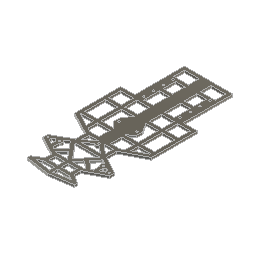
carBodyFrontEnd v1 (Autodesk Fusion 360 design; units mm, degrees)
Autodesk Fusion 360 part; units mm, degrees
(part 1 of 2)
sketch "v0.1" plane through (0, 0, 0) normal (0, 0, 1) x (1, 0, 0)
  line L0 (-45, 50) -> (37, 50)
  line L1 (37, 50) -> (37, 134)
  line L2 (37, 134) -> (-45, 134)
  line L3 (-45, 134) -> (-45, 50)
  line L4 (-69, 50) -> (61, 50)
  line L5 (61, 50) -> (61, -28)
  line L6 (61, -28) -> (-69, -28)
  line L7 (-69, -28) -> (-69, 50)
  line L8 (-30.5, -48) -> (22.5, -48)
  line L9 (22.5, -48) -> (22.5, -65)
  line L10 (22.5, -65) -> (-30.5, -65)
  line L11 (-30.5, -65) -> (-30.5, -48)
  line L12 (-60.5, -82) -> (52.5, -82)
  line L13 (52.5, -82) -> (52.5, -90)
  line L14 (52.5, -90) -> (-60.5, -90)
  line L15 (-60.5, -90) -> (-60.5, -82)
  line L16 (-30.5002, -118) -> (22.4998, -118)
  line L17 (22.4998, -118) -> (22.4998, -107)
  line L18 (22.4998, -107) -> (-30.5002, -107)
  line L19 (-30.5002, -107) -> (-30.5002, -118)
  line L20 (-44.0003, -127.9997) -> (35.9997, -127.9997)
  line L21 (35.9997, -127.9997) -> (35.9997, -132.9997)
  line L22 (35.9997, -132.9997) -> (-44.0003, -132.9997)
  line L23 (-44.0003, -132.9997) -> (-44.0003, -127.9997)
  circle A0 centre (-4.0003, -130.4997) radius 1.6
  circle A1 centre (1.9997, -130.4997) radius 1.6
  circle A2 centre (-10.0003, -130.4997) radius 1.6
  circle A3 centre (-18.0003, -130.4997) radius 1.6
  circle A4 centre (9.9997, -130.4997) radius 1.6
  line L24 (-10.0003, -128.8997) -> (-18.0003, -128.8997)
  line L25 (-10.0003, -132.0997) -> (-18.0003, -132.0997)
  line L26 (1.9997, -128.8997) -> (9.9997, -128.8997)
  line L27 (9.9997, -132.0997) -> (1.9997, -132.0997)
  line L28 (-45, 128.75) -> (-45, 134)
  line L29 (-45, 134) -> (-39.1, 134)
  line L30 (37, 134) -> (31, 134)
  line L31 (31, 134) -> (31, 130)
  line L32 (31, 130) -> (37, 130)
  line L33 (37, 130) -> (37, 134)
  line L34 (-45, 134) -> (-39, 134)
  line L35 (-39, 134) -> (-39, 130)
  line L36 (-39, 130) -> (-45, 130)
  line L37 (-45, 130) -> (-45, 134)
  circle A5 centre (-39, 130) radius 1.6
  circle A6 centre (31, 130) radius 1.6
  circle A7 centre (4.25, 87.9939) radius 1.6
  circle A8 centre (-11.75, 88.0061) radius 1.6
  line L38 (-11.75, 88.0061) -> (-17.75, 88.0107)
  circle A9 centre (-17.75, 88.0107) radius 1.6
  line L39 (4.25, 87.9939) -> (10.25, 87.9939)
  circle A10 centre (10.25, 87.9939) radius 1.6
  line L40 (10.25, 87.9939) -> (20.25, 87.9939)
  circle A11 centre (20.25, 87.9939) radius 1.6
  line L41 (-17.75, 88.0107) -> (-27.75, 88.0184)
  circle A12 centre (-27.75, 88.0184) radius 1.6
  line L42 (-27.7488, 89.6184) -> (-17.7488, 89.6107)
  line L43 (-27.7512, 86.4184) -> (-17.7512, 86.4107)
  line L44 (10.25, 89.5939) -> (20.25, 89.5939)
  line L45 (20.25, 86.3939) -> (10.25, 86.3939)
  line L46 (-69, 50) -> (-57.5, 50)
  line L47 (-57.5, 50) -> (-57.5, 45)
  line L48 (-57.5, 45) -> (-69, 45)
  line L49 (-69, 45) -> (-69, 50)
  circle A13 centre (-57.5, 45) radius 1.6
  line L50 (-57.5, 45) -> (-57.5, 32)
  circle A14 centre (-57.5, 32) radius 1.6
  line L51 (-55.9, 45.0023) -> (-55.9, 32)
  line L52 (-59.1, 45) -> (-59.1, 32)
  line L53 (61, 50) -> (49.5, 50)
  line L54 (49.5, 50) -> (49.5, 45)
  line L55 (49.5, 45) -> (61, 45)
  line L56 (61, 45) -> (61, 50)
  circle A15 centre (49.5, 45) radius 1.6
  line L57 (49.5, 45) -> (49.5, 32)
  circle A16 centre (49.5, 32) radius 1.6
  line L58 (51.1, 45) -> (51.1, 32)
  line L59 (47.9, 32) -> (47.9, 45)
  line L60 (-57.5, 45) -> (-57.5, -26)
  circle A17 centre (-57.5, -26) radius 1.6
  line L61 (49.5, 45) -> (49.5, -26)
  circle A18 centre (49.5, -26) radius 1.6
  circle A19 centre (-4, -51.9) radius 1.6
  circle A20 centre (33.037, -81.135) radius 1.6
  circle A21 centre (-41.033, -81.1414) radius 1.6
  line L62 (22.5, -48) -> (61, -28)
  line L63 (-30.5, -48) -> (-69, -28)
  line L64 (-60.5, -82) -> (-30.5, -65)
  line L65 (22.5, -65) -> (52.5, -82)
  line L66 (22.4998, -107) -> (52.5, -90)
  line L67 (-30.5002, -107) -> (-60.5, -90)
  line L68 (4.25, 87.9939) -> (-11.75, 88.0061)
  line L69 (-4, 134) -> (-3.75, 88)
  line L70 (-44.0003, -127.9997) -> (-30.5002, -118)
  line L71 (35.9997, -127.9997) -> (22.4998, -118)
  line L72 (-4.0003, -132.9997) -> (-4.0003, -138.9997)
  line L73 (-44.0003, -132.9997) -> (-4.0003, -138.9997)
  line L74 (-4.0003, -138.9997) -> (35.9997, -132.9997)
  line L75 (-4.0003, -130.4997) -> (1.9997, -130.4997)
  line L76 (-4.0003, -130.4997) -> (-10.0003, -130.4997)
  line L77 (-4, -65) -> (-4, -83)
  line L78 (-4, -83) -> (-4, -86)
  line L79 (-4, -86) -> (-56, -86)
  line L80 (-4, -86) -> (48, -86)
  circle A22 centre (48, -86) radius 1.1
  circle A23 centre (-56, -86) radius 1.1
  line L81 (20.25, 87.9939) -> (37, 87.9939)
  line L82 (-27.75, 88.0184) -> (-45, 88.0184)
  line L83 (37, 50) -> (24, 50)
  line L84 (24, 50) -> (24, 110)
  line L85 (24, 110) -> (37, 110)
  line L86 (37, 110) -> (37, 50)
  line L87 (-45, 50) -> (-32, 50)
  line L88 (-32, 50) -> (-32, 110)
  line L89 (-32, 110) -> (-45, 110)
  line L90 (-45, 110) -> (-45, 50)
  line L91 (37, 110) -> (31, 110)
  line L92 (31, 110) -> (31, 50)
  line L93 (31, 50) -> (37, 50)
  line L94 (37, 50) -> (37, 110)
  line L95 (-45, 110) -> (-39, 110)
  line L96 (-39, 110) -> (-39, 50)
  line L97 (-39, 50) -> (-45, 50)
  line L98 (-45, 50) -> (-45, 110)
  line L99 (24, 110) -> (27, 110)
  line L100 (27, 110) -> (27, 105)
  line L101 (27, 105) -> (24, 105)
  line L102 (24, 105) -> (24, 110)
  circle A24 centre (27, 105) radius 1.6
  circle A25 centre (27, 88.3333) radius 1.6
  circle A26 centre (27, 71.6667) radius 1.6
  circle A27 centre (27, 55) radius 1.6
  line L103 (-32, 110) -> (-35, 110)
  line L104 (-35, 110) -> (-35, 105)
  line L105 (-35, 105) -> (-32, 105)
  line L106 (-32, 105) -> (-32, 110)
  circle A28 centre (-35, 105) radius 1.6
  circle A29 centre (-35, 88.3333) radius 1.6
  circle A30 centre (-35, 71.6667) radius 1.6
  circle A31 centre (-35, 55) radius 1.6
  line L107 (-69, -28) -> (-49.75, -28)
  line L108 (-49.75, -28) -> (-49.75, -18)
  line L109 (-49.75, -18) -> (-69, -18)
  line L110 (-69, -18) -> (-69, -28)
  line L111 (-69, -18) -> (61, -18)
  line L112 (61, -18) -> (61, 17)
  line L113 (61, 17) -> (-69, 17)
  line L114 (-69, 17) -> (-69, -18)
  line L115 (-69, 17) -> (-55, 17)
  line L116 (-55, 17) -> (-55, 10)
  line L117 (-55, 10) -> (-69, 10)
  line L118 (-69, 10) -> (-69, 17)
  line L119 (61, 17) -> (47, 17)
  line L120 (47, 17) -> (47, 10)
  line L121 (47, 10) -> (61, 10)
  line L122 (61, 10) -> (61, 17)
  circle A32 centre (-55, 10) radius 1.6
  circle A33 centre (-21, 10) radius 1.6
  circle A34 centre (13, 10) radius 1.6
  circle A35 centre (47, 10) radius 1.6
  circle A36 centre (-55, -11) radius 1.6
  circle A37 centre (-21, -11) radius 1.6
  circle A38 centre (13, -11) radius 1.6
  circle A39 centre (47, -11) radius 1.6
  line L123 (-69, 17) -> (61, 17)
  line L124 (61, 17) -> (61, 18)
  line L125 (61, 18) -> (-69, 18)
  line L126 (-69, 18) -> (-69, 17)
  line L127 (61, 18) -> (-69, 18)
  line L128 (-69, 18) -> (-69, 23)
  line L129 (-69, 23) -> (61, 23)
  line L130 (61, 23) -> (61, 18)
  circle A40 centre (18.0038, -78.6409) radius 1.6
  circle A41 centre (18.0038, -78.6409) radius 5
  circle A42 centre (-25.9962, -78.6409) radius 5
  circle A43 centre (-25.9962, -78.6409) radius 1.6
  dimension "d1" = 82
  dimension "d2" = 84
  dimension "d3" = 78
  dimension "d4" = 130
  dimension "d6" = 17
  dimension "d11" = 113
  dimension "d12" = 8
  dimension "d15" = 11
  dimension "d16" = 53
  dimension "d20" = 80
  dimension "d21" = 5
  dimension "d25" = 3.2
  dimension "d29" = 3.2
  dimension "d31" = 3.2
  dimension "d32" = 3.2
  dimension "d35" = 3.2
  dimension "d38" = 6
  dimension "d39" = 4
  dimension "d42" = 6
  dimension "d43" = 4
  dimension "d44" = 3.2
  dimension "d45" = 3.2
  dimension "d53" = 3.2
  dimension "d54" = 3.2
  dimension "d55" = 6
  dimension "d56" = 3.2
  dimension "d58" = 6
  dimension "d59" = 3.2
  dimension "d60" = 10
  dimension "d61" = 3.2
  dimension "d62" = 10
  dimension "d63" = 3.2
  dimension "d64" = 11.5
  dimension "d65" = 3.2
  dimension "d66" = 13
  dimension "d67" = 3.2
  dimension "d68" = 11.5
  dimension "d69" = 5
  dimension "d70" = 5
  dimension "d71" = 3.2
  dimension "d72" = 13
  dimension "d73" = 3.2
  dimension "d74" = 71
  dimension "d75" = 3.2
  dimension "d77" = 71
  dimension "d78" = 3.2
  dimension "d80" = 3.2
  dimension "d83" = 3.2
  dimension "d84" = 3.2
  dimension "d90" = 53
  dimension "d92" = 46
  dimension "d93" = 16
  dimension "d95" = 6
  dimension "d99" = 6
  dimension "d100" = 6
  dimension "d101" = 8
  dimension "d102" = 8
  dimension "d108" = 52
  dimension "d109" = 52
  dimension "d110" = 2.2
  dimension "d111" = 2.2
  dimension "d112" = 13
  dimension "d113" = 60
  dimension "d114" = 13
  dimension "d115" = 60
  dimension "d116" = 60
  dimension "d117" = 6
  dimension "d118" = 60
  dimension "d119" = 3
  dimension "d120" = 5
  dimension "d121" = 3.2
  dimension "d124" = 0
  dimension "d125" = -50
  dimension "d126" = 3
  dimension "d127" = 5
  dimension "d128" = 3.2
  dimension "d131" = 0
  dimension "d132" = -50
  dimension "d133" = 10
  dimension "d134" = 35
  dimension "d135" = 14
  dimension "d136" = 7
  dimension "d137" = 14
  dimension "d138" = 7
  dimension "d139" = 3.2
  dimension "d142" = 102
  dimension "d143" = -21
  dimension "d144" = 1
  dimension "d145" = 130
  dimension "d146" = 5
  dimension "d154" = 3.2
  dimension "d155" = 10
  dimension "d156" = 3.2
  dimension "d157" = 10
  constraint horizontal L0
  constraint vertical L1
  constraint horizontal L2
  constraint vertical L3
  constraint horizontal L4
  constraint vertical L5
  constraint horizontal L6
  constraint vertical L7
  constraint horizontal L8
  constraint vertical L9
  constraint horizontal L10
  constraint vertical L11
  constraint horizontal L12
  constraint vertical L13
  constraint horizontal L14
  constraint vertical L15
  constraint horizontal L16
  constraint vertical L17
  constraint horizontal L18
  constraint vertical L19
  constraint vertical L21
  constraint horizontal L22
  constraint vertical L23
  constraint coincident A2 L24.start
  constraint coincident A3 L24.end
  constraint tangent A3 L24
  constraint coincident A2 L25.start
  constraint coincident A3 L25.end
  constraint tangent A3 L25
  constraint coincident A1 L26.start
  constraint coincident A4 L26.end
  constraint tangent A4 L26
  constraint coincident A4 L27.start
  constraint coincident A1 L27.end
  constraint tangent A1 L27
  constraint vertical L28
  constraint horizontal L29
  constraint horizontal L30
  constraint vertical L31
  constraint horizontal L32
  constraint vertical L33
  constraint horizontal L34
  constraint vertical L35
  constraint horizontal L36
  constraint vertical L37
  constraint coincident L35.end L36.start
  constraint coincident L31.end L32.start
  constraint coincident A8.centre L38.start
  constraint coincident L38.end A9.centre
  constraint coincident A7.centre L39.start
  constraint coincident L39.end A10.centre
  constraint coincident L40.end A11.centre
  constraint coincident L41.end A12.centre
  constraint coincident A12 L42.start
  constraint coincident A9 L42.end
  constraint tangent A9 L42
  constraint coincident A12 L43.start
  constraint coincident A9 L43.end
  constraint tangent A9 L43
  constraint coincident A10 L44.start
  constraint coincident A11 L44.end
  constraint tangent A11 L44
  constraint coincident A11 L45.start
  constraint coincident A10 L45.end
  constraint tangent A10 L45
  constraint horizontal L46
  constraint vertical L47
  constraint horizontal L48
  constraint vertical L49
  constraint coincident L47.end L48.start
  constraint perpendicular L48 L50
  constraint coincident L50.end A14.centre
  constraint coincident A13 L51.start
  constraint coincident A14 L51.end
  constraint tangent A14 L51
  constraint parallel L47 L51
  constraint coincident A13 L52.start
  constraint coincident L48 L52.start
  constraint coincident A14 L52.end
  constraint tangent A14 L52
  constraint horizontal L53
  constraint vertical L54
  constraint horizontal L55
  constraint vertical L56
  constraint coincident L54.end L55.start
  constraint perpendicular L55 L57
  constraint coincident L57.end A16.centre
  constraint coincident A15 L58.start
  constraint coincident L55 L58.start
  constraint coincident A16 L58.end
  constraint tangent A16 L58
  constraint coincident A16 L59.start
  constraint coincident A15 L59.end
  constraint tangent A15 L59
  constraint parallel L50 L60
  constraint coincident L60.end A17.centre
  constraint perpendicular L55 L61
  constraint coincident L61.end A18.centre
  constraint midpoint L2 L69.start
  constraint midpoint L68 L69.end
  constraint tangent A10 L44
  constraint tangent A11 L45
  constraint tangent A12 L42
  constraint tangent A12 L43
  constraint midpoint L22 L72.start
  constraint perpendicular L22 L72
  constraint coincident A0.centre L75.start
  constraint coincident A1.centre L75.end
  constraint coincident A2.centre L76.end
  constraint tangent A2 L24
  constraint tangent A2 L25
  constraint tangent A1 L26
  constraint tangent A4 L27
  constraint midpoint L10 L77.start
  constraint perpendicular L78 L79
  constraint perpendicular L78 L80
  constraint coincident L80.end A22.centre
  constraint coincident L79.end A23.centre
  constraint coincident L1 L81.end
  constraint perpendicular L1 L81
  constraint coincident L3 L82.end
  constraint perpendicular L3 L82
  constraint horizontal L83
  constraint vertical L84
  constraint horizontal L85
  constraint vertical L86
  constraint horizontal L87
  constraint vertical L88
  constraint horizontal L89
  constraint vertical L90
  constraint horizontal L91
  constraint vertical L92
  constraint horizontal L93
  constraint vertical L94
  constraint horizontal L95
  constraint vertical L96
  constraint horizontal L97
  constraint vertical L98
  constraint horizontal L99
  constraint vertical L100
  constraint horizontal L101
  constraint vertical L102
  constraint coincident L100.end L101.start
  constraint horizontal L103
  constraint vertical L104
  constraint horizontal L105
  constraint vertical L106
  constraint coincident L104.end L105.start
  constraint horizontal L107
  constraint vertical L108
  constraint horizontal L109
  constraint vertical L110
  constraint horizontal L111
  constraint vertical L112
  constraint horizontal L113
  constraint vertical L114
  constraint horizontal L115
  constraint vertical L116
  constraint horizontal L117
  constraint vertical L118
  constraint horizontal L119
  constraint vertical L120
  constraint horizontal L121
  constraint vertical L122
  constraint coincident L116.end L117.start
  constraint horizontal L123
  constraint vertical L124
  constraint horizontal L125
  constraint vertical L126
  constraint coincident L5 L124.end
  constraint horizontal L127
  constraint vertical L128
  constraint horizontal L129
  constraint vertical L130
  constraint concentric A40 A41
  constraint concentric A42 A43
  measures "d1" distance of L1.end L2.end
  measures "d2" distance of L0.start L2.end
  measures "d3" distance of L4.end L5.end
  measures "d4" distance of L5.end L6.end
  measures "d6" distance of L8.start L10.end
  measures "d11" distance of L12.start L12.end
  measures "d12" distance of L12.start L14.end
  measures "d15" distance of L16.start L18.end
  measures "d16" distance of L17.end L18.end
  measures "d20" distance of L20.start L20.end
  measures "d21" distance of L20.start L22.end
  measures "d25" diameter of A0
  measures "d29" diameter of A1
  measures "d31" diameter of A2
  measures "d32" diameter of A3
  measures "d35" diameter of A4
  measures "d38" distance of L1.end L30.end
  measures "d39" distance of L1.end L32.end
  measures "d42" distance of L2.end L34.end
  measures "d43" distance of L2.end L36.end
  measures "d44" diameter of A5
  measures "d45" diameter of A6
  measures "d53" diameter of A7
  measures "d54" diameter of A8
  measures "d55" distance of A8.centre L38.end
  measures "d56" diameter of A9
  measures "d58" distance of A7.centre L39.end
  measures "d59" diameter of A10
  measures "d60" distance of L39.end L40.end
  measures "d61" diameter of A11
  measures "d62" distance of L38.end L41.end
  measures "d63" diameter of A12
  measures "d64" distance of L4.start L46.end
  measures "d65" diameter of A13
  measures "d66" distance of L47.end L50.end
  measures "d67" diameter of A14
  measures "d68" distance of L4.end L53.end
  measures "d69" distance of L4.end L55.end
  measures "d70" distance of L4.start L48.end
  measures "d71" diameter of A15
  measures "d72" distance of L54.end L57.end
  measures "d73" diameter of A16
  measures "d74" distance of L47.end L60.end
  measures "d75" diameter of A17
  measures "d77" distance of L54.end L61.end
  measures "d78" diameter of A18
  measures "d80" diameter of A19
  measures "d83" diameter of A20
  measures "d84" diameter of A21
  measures "d90" distance of L8.start L8.end
  measures "d92" vertical distance of L69.start L69.end
  measures "d93" horizontal distance of A7.centre A8.centre
  measures "d95" distance of L72.start L72.end
  measures "d99" distance of A0.centre A1.centre
  measures "d100" distance of A0.centre A2.centre
  measures "d101" distance of L24.start L24.end
  measures "d102" distance of L26.start L26.end
  measures "d108" distance of L78.end L79.end
  measures "d109" distance of L78.end L80.end
  measures "d110" diameter of A22
  measures "d111" diameter of A23
  measures "d112" distance of L0.end L83.end
  measures "d113" distance of L0.end L85.end
  measures "d114" distance of L0.start L87.end
  measures "d115" distance of L0.start L89.end
  measures "d116" distance of L85.end L0.end
  measures "d117" distance of L89.end L95.end
  measures "d118" distance of L89.end L0.start
  measures "d119" distance of L84.end L99.end
  measures "d120" distance of L84.end L101.end
  measures "d121" diameter of A24
  measures "d126" distance of L88.end L103.end
  measures "d127" distance of L88.end L105.end
  measures "d128" diameter of A28
  measures "d133" distance of L6.end L109.end
  measures "d134" distance of L109.end L113.end
  measures "d135" distance of L113.end L115.end
  measures "d136" distance of L113.end L117.end
  measures "d137" distance of L112.end L119.end
  measures "d138" distance of L112.end L121.end
  measures "d139" diameter of A32
  measures "d144" distance of L113.end L125.end
  measures "d145" distance of L124.end L125.end
  measures "d146" distance of L124.end L129.end
  measures "d154" diameter of A40
  measures "d155" diameter of A41
  measures "d156" diameter of A43
  measures "d157" diameter of A42
sketch "v0.2" plane through (0, 0, 0) normal (0, 0, 1) x (1, 0, 0)
  circle A0 centre (-4, -51.9) radius 1.65
  line L0 (-30.5, -48) -> (22.5, -48)
  circle A1 centre (-56, -86) radius 1.1
  line L1 (-69, -28) -> (-69, 50)
  line L2 (61, 50) -> (61, -28)
  line L3 (22.5, -48) -> (61, -28)
  line L4 (-30.5, -65) -> (-30.5, -48)
  line L5 (22.5, -65) -> (-30.5, -65)
  line L6 (22.5, -48) -> (22.5, -65)
  line L7 (-30.5, -48) -> (-69, -28)
  line L8 (35.9997, -127.9997) -> (35.9997, -132.9997)
  circle A2 centre (33.037, -81.135) radius 1.65
  line L9 (-45, 50) -> (37, 50)
  line L10 (-4, -86) -> (48, -86)
  line L11 (-45, 110) -> (-45, 50)
  line L12 (-4.0003, -138.9997) -> (35.9997, -132.9997)
  line L13 (-45, 134) -> (-45, 50)
  line L14 (-69, 50) -> (61, 50)
  line L15 (-4, -86) -> (-56, -86)
  line L16 (-4, -65) -> (-4, -83)
  line L17 (37, 110) -> (37, 50)
  line L18 (24, 50) -> (24, 110)
  line L19 (-39, 50) -> (-45, 50)
  line L20 (31, 110) -> (31, 50)
  line L21 (22.5, -65) -> (52.5, -82)
  line L22 (52.5, -90) -> (-60.5, -90)
  line L23 (-60.5, -82) -> (52.5, -82)
  line L24 (-32, 50) -> (-32, 110)
  line L25 (52.5, -82) -> (52.5, -90)
  line L26 (37, 134) -> (-45, 134)
  line L27 (37, 50) -> (37, 110)
  line L28 (-39, 110) -> (-39, 50)
  line L29 (37, 50) -> (37, 134)
  line L30 (-4, -83) -> (-4, -86)
  line L31 (-60.5, -82) -> (-30.5, -65)
  circle A3 centre (48, -86) radius 1.1
  line L32 (-45, 50) -> (-45, 110)
  line L33 (-32, 110) -> (-45, 110)
  line L34 (-45, 128.75) -> (-45, 134)
  line L35 (-35, 110) -> (-35, 105)
  line L36 (24, 110) -> (37, 110)
  line L37 (31, 50) -> (37, 50)
  line L38 (27, 110) -> (27, 105)
  line L39 (-35, 105) -> (-32, 105)
  line L40 (4.25, 87.9939) -> (10.25, 87.9939)
  circle A4 centre (-35, 55) radius 1.6
  line L41 (-45, 134) -> (-39.1, 134)
  line L42 (-32, 105) -> (-32, 110)
  line L43 (27, 105) -> (24, 105)
  circle A5 centre (27, 88.3333) radius 1.6
  circle A6 centre (27, 105) radius 1.6
  line L44 (-45, 50) -> (-32, 50)
  line L45 (24, 110) -> (27, 110)
  line L46 (-45, 110) -> (-39, 110)
  circle A7 centre (27, 71.6667) radius 1.6
  line L47 (37, 50) -> (24, 50)
  circle A8 centre (27, 55) radius 1.6
  circle A9 centre (-35, 88.3333) radius 1.6
  circle A10 centre (-35, 71.6667) radius 1.6
  line L48 (-32, 110) -> (-35, 110)
  line L49 (37, 110) -> (31, 110)
  circle A11 centre (-35, 105) radius 1.6
  line L50 (24, 105) -> (24, 110)
  line L51 (-60.5, -90) -> (-60.5, -82)
  circle A12 centre (-41.033, -81.1414) radius 1.65
  line L52 (-4.0003, -132.9997) -> (-4.0003, -138.9997)
  line L53 (-44.0003, -132.9997) -> (-4.0003, -138.9997)
  line L54 (-44.0003, -132.9997) -> (-44.0003, -127.9997)
  line L55 (20.4998, -118) -> (-28.5002, -118)
  line L56 (-28.5002, -118) -> (-28.5002, -107)
  line L57 (-28.5002, -107) -> (20.4998, -107)
  line L58 (20.4998, -107) -> (20.4998, -118)
  line L59 (35.9997, -127.9997) -> (20.4998, -118)
  line L60 (-44.0003, -127.9997) -> (-28.5002, -118)
  line L61 (20.4998, -107) -> (52.5, -90)
  line L62 (-28.5002, -107) -> (-60.5, -90)
  line L63 (52.5, -90) -> (44.5, -90)
  line L64 (44.5, -90) -> (44.5, -82)
  line L65 (44.5, -82) -> (52.5, -82)
  line L66 (52.5, -82) -> (52.5, -90)
  line L67 (-60.5, -82) -> (-52.5, -82)
  line L68 (-52.5, -82) -> (-52.5, -90)
  line L69 (-52.5, -90) -> (-60.5, -90)
  line L70 (-60.5, -90) -> (-60.5, -82)
  line L71 (-34.4973, -103.814) -> (-31.6823, -98.5153)
  line L72 (-44.5001, -98.5) -> (-41.6852, -93.2013)
  line L73 (-28.5002, -118) -> (-22.5002, -118)
  line L74 (-22.5002, -118) -> (-22.5002, -107)
  line L75 (-22.5002, -107) -> (-28.5002, -107)
  line L76 (-28.5002, -107) -> (-28.5002, -118)
  line L77 (20.4998, -118) -> (14.4998, -118)
  line L78 (14.4998, -118) -> (14.4998, -107)
  line L79 (14.4998, -107) -> (20.4998, -107)
  line L80 (20.4998, -107) -> (20.4998, -118)
  line L81 (-41.6852, -93.2013) -> (-52.5, -87.4559)
  line L82 (20.4998, -107) -> (-28.5002, -107)
  line L83 (-28.5002, -107) -> (-28.5002, -101)
  line L84 (-28.5002, -101) -> (20.4998, -101)
  line L85 (20.4998, -101) -> (20.4998, -107)
  line L86 (42.9588, -95.0687) -> (40.1439, -89.77)
  line L87 (40.1439, -89.77) -> (44.5, -87.4558)
  line L88 (-31.6823, -98.5153) -> (-27.0054, -101)
  line L89 (22.5, -65) -> (-30.5, -65)
  line L90 (-30.5, -65) -> (-30.5, -71)
  line L91 (-30.5, -71) -> (22.5, -71)
  line L92 (22.5, -71) -> (22.5, -65)
  line L93 (41.4913, -75.7617) -> (38.5332, -80.9819)
  line L94 (-41.4357, -71.1969) -> (-38.4777, -76.4171)
  line L95 (33.9769, -71.5036) -> (31.0189, -76.7237)
  line L96 (-49.8898, -75.9876) -> (-46.9317, -81.2077)
  line L97 (38.5332, -80.9819) -> (31.0189, -76.7237)
  line L98 (-38.4777, -76.4171) -> (-46.9317, -81.2077)
  line L99 (-38.4777, -76.4171) -> (-28.9182, -71)
  line L100 (38.5332, -80.9819) -> (44.5, -84.363)
  line L101 (31.0189, -76.7237) -> (20.9182, -71)
  line L102 (-46.9317, -81.2077) -> (-52.5, -84.363)
  circle A13 centre (33.037, -81.135) radius 5
  circle A14 centre (-41.033, -81.1414) radius 5
  line L103 (-36.033, -86.1414) -> (-46.033, -86.1414)
  line L104 (-46.033, -86.1414) -> (-46.033, -76.1414)
  line L105 (-46.033, -76.1414) -> (-36.033, -76.1414)
  line L106 (-36.033, -76.1414) -> (-36.033, -86.1414)
  line L107 (-36.033, -76.1414) -> (-46.033, -86.1414)
  line L108 (-44.5685, -84.677) -> (-47.6377, -81.6078)
  line L109 (-37.4975, -77.6059) -> (-38.6108, -76.4925)
  line L110 (-41.033, -86.1414) -> (-44.033, -86.1414)
  line L111 (-41.033, -86.1414) -> (-38.033, -86.1414)
  line L112 (-38.033, -86.1414) -> (-38.033, -95.1415)
  line L113 (-44.033, -86.1414) -> (-44.033, -91.954)
  line L114 (38.037, -86.135) -> (28.037, -86.135)
  line L115 (28.037, -86.135) -> (28.037, -76.135)
  line L116 (28.037, -76.135) -> (38.037, -76.135)
  line L117 (38.037, -76.135) -> (38.037, -86.135)
  line L118 (38.037, -86.135) -> (28.037, -76.135)
  line L119 (36.5725, -84.6705) -> (39.6362, -81.6069)
  line L120 (29.5015, -77.5995) -> (30.6093, -76.4916)
  line L121 (33.037, -86.135) -> (30.037, -86.135)
  line L122 (33.037, -86.135) -> (36.037, -86.135)
  line L123 (36.037, -86.135) -> (36.037, -91.9518)
  line L124 (30.037, -86.135) -> (30.037, -95.1392)
  line L125 (-4.0002, -118) -> (-7.0002, -118)
  line L126 (-7.0002, -118) -> (-7.0002, -107)
  line L127 (-7.0002, -107) -> (-4.0002, -107)
  line L128 (-4.0002, -107) -> (-4.0002, -118)
  line L129 (-4.0002, -118) -> (-1.0002, -118)
  line L130 (-1.0002, -118) -> (-1.0002, -107)
  line L131 (-1.0002, -107) -> (-4.0002, -107)
  line L132 (-4.0002, -107) -> (-4.0002, -118)
  line L133 (20.4998, -118) -> (-28.5002, -118)
  line L134 (-28.5002, -118) -> (-28.5002, -124)
  line L135 (-28.5002, -124) -> (20.4998, -124)
  line L136 (20.4998, -124) -> (20.4998, -118)
  line L137 (22.5, -48) -> (-30.5, -48)
  line L138 (-30.5, -48) -> (-30.5, -42)
  line L139 (-30.5, -42) -> (22.5, -42)
  line L140 (22.5, -42) -> (22.5, -48)
  line L141 (22.5, -65) -> (16.5, -65)
  line L142 (16.5, -65) -> (16.5, -48)
  line L143 (16.5, -48) -> (22.5, -48)
  line L144 (22.5, -48) -> (22.5, -65)
  line L145 (-30.5, -65) -> (-24.5, -65)
  line L146 (-24.5, -65) -> (-24.5, -48)
  line L147 (-24.5, -48) -> (-30.5, -48)
  line L148 (-30.5, -48) -> (-30.5, -65)
  line L149 (-4, -48) -> (-10, -48)
  line L150 (-4, -48) -> (2, -48)
  line L151 (16.5, -65) -> (-4, -48)
  line L152 (7.4381, -57.4852) -> (5.5231, -59.7945)
  line L153 (7.4381, -57.4852) -> (9.3531, -55.176)
  line L154 (5.5231, -59.7945) -> (11.8003, -65)
  line L155 (9.3531, -55.176) -> (16.5, -61.1027)
  line L156 (9.3531, -55.176) -> (0.6997, -48)
  line L157 (5.5231, -59.7945) -> (-4, -51.8973)
  line L158 (-4, -48) -> (-24.5, -65)
  line L159 (-15.9609, -57.9188) -> (-17.8759, -55.6095)
  line L160 (-15.9609, -57.9188) -> (-14.0459, -60.2281)
  line L161 (-14.0459, -60.2281) -> (-19.8003, -65)
  line L162 (-17.8759, -55.6095) -> (-24.5, -61.1027)
  line L163 (-17.8759, -55.6095) -> (-8.6997, -48)
  line L164 (-14.0459, -60.2281) -> (-4, -51.8973)
  circle A15 centre (-4, -51.9) radius 5
  line L165 (-4.0002, -101) -> (20.9182, -71)
  line L166 (-4.0002, -101) -> (-28.9182, -71)
  line L167 (9.237, -85.0633) -> (6.9292, -83.1464)
  line L168 (11.1299, -82.7843) -> (13.4377, -84.7012)
  line L169 (13.4377, -84.7012) -> (-0.1003, -101)
  line L170 (6.9292, -83.1464) -> (-4.0002, -96.3047)
  line L171 (6.9292, -83.1464) -> (17.0183, -71)
  line L172 (13.4377, -84.7012) -> (23.5699, -72.5027)
  line L173 (-15.5316, -87.1168) -> (-17.8394, -89.0336)
  line L174 (-20.2247, -81.4665) -> (-17.9169, -79.5497)
  line L175 (-17.9169, -79.5497) -> (-4.0002, -96.3047)
  line L176 (-17.9169, -79.5497) -> (-25.0183, -71)
  line L177 (-17.8394, -89.0336) -> (-7.9001, -101)
  line L178 (-17.8394, -89.0336) -> (-31.5699, -72.5027)
  line L179 (-27.0054, -101) -> (-38.033, -95.1415)
  line L180 (-41.6852, -93.2013) -> (-38.033, -95.1415)
  line L181 (-32.5192, -98.0707) -> (-19.3905, -87.1661)
  line L182 (-30.0239, -95.9982) -> (-31.9408, -93.6904)
  line L183 (-31.9408, -93.6904) -> (-35.3829, -96.5494)
  line L184 (-31.9408, -93.6904) -> (-21.3073, -84.8583)
  line L185 (40.1439, -89.77) -> (30.037, -95.1392)
  line L186 (30.037, -95.1392) -> (19.0049, -101)
  line L187 (24.521, -98.0696) -> (11.3918, -87.1643)
  line L188 (18.2376, -92.8506) -> (16.3208, -95.1583)
  line L189 (18.2376, -92.8506) -> (20.1545, -90.5428)
  line L190 (20.1545, -90.5428) -> (27.3846, -96.5483)
  line L191 (16.3208, -95.1583) -> (21.6573, -99.5909)
  line L192 (16.3208, -95.1583) -> (9.4749, -89.472)
  line L193 (20.1545, -90.5428) -> (13.3086, -84.8565)
  line L194 (-27.4733, -93.8796) -> (-25.5565, -96.1874)
  line L195 (-25.5565, -96.1874) -> (-30.221, -100.0617)
  line L196 (-25.5565, -96.1874) -> (-17.4737, -89.4738)
  line L197 (30.037, -86.135) -> (30.037, -85.135)
  line L198 (36.037, -86.135) -> (36.037, -85.135)
  line L199 (-38.033, -86.1414) -> (-38.033, -85.1414)
  line L200 (-44.033, -86.1414) -> (-44.033, -85.1414)
  line L201 (-4.0002, -101) -> (-4.0002, -96.3047)
  line L202 (-4.0002, -96.3047) -> (-9.2369, -90)
  line L203 (-9.2369, -90) -> (-13.1368, -90)
  line L204 (-13.1368, -90) -> (-4.0002, -101)
  line L205 (52.5, -90) -> (43.5, -90)
  line L206 (43.5, -90) -> (43.5, -82)
  line L207 (43.5, -82) -> (52.5, -82)
  line L208 (52.5, -82) -> (52.5, -90)
  line L209 (-60.5, -90) -> (-51.5, -90)
  line L210 (-51.5, -90) -> (-51.5, -82)
  line L211 (-51.5, -82) -> (-60.5, -82)
  line L212 (-60.5, -82) -> (-60.5, -90)
  line L213 (-69, -28) -> (-63, -28)
  line L214 (-63, -28) -> (-63, 50)
  line L215 (-63, 50) -> (-69, 50)
  line L216 (-69, 50) -> (-69, -28)
  line L217 (61, -28) -> (55, -28)
  line L218 (55, -28) -> (55, 50)
  line L219 (55, 50) -> (61, 50)
  line L220 (61, 50) -> (61, -28)
  line L221 (-57.2963, -34.0798) -> (-54.5304, -28.7554)
  line L222 (-47.539, -39.1486) -> (-44.7731, -33.8241)
  line L223 (-54.5304, -28.7554) -> (-44.7731, -33.8241)
  line L224 (-44.7731, -33.8241) -> (-29.0345, -42)
  line L225 (-54.5304, -28.7554) -> (-63, -24.3556)
  line L226 (42.8853, -37.4102) -> (40.1193, -32.0858)
  line L227 (40.1193, -32.0858) -> (55, -24.3556)
  line L228 (40.1193, -32.0858) -> (21.0345, -42)
  line L229 (-69, 50) -> (61, 50)
  line L230 (61, 50) -> (61, 44)
  line L231 (61, 44) -> (-69, 44)
  line L232 (-69, 44) -> (-69, 50)
  line L233 (-4, -42) -> (-14, -42)
  line L234 (-14, -42) -> (-14, 44)
  line L235 (-14, 44) -> (-4, 44)
  line L236 (-4, -42) -> (6, -42)
  line L237 (6, -42) -> (6, 44)
  line L238 (6, 44) -> (-4, 44)
  line L239 (-69, -2.4999) -> (61, -2.4999)
  line L240 (-14, 44) -> (-63, 44)
  line L241 (6, 44) -> (55, 44)
  line L242 (30.5, 44) -> (33.5, 44)
  line L243 (30.5, 44) -> (27.5, 44)
  line L244 (-38.5, 44) -> (-35.5, 44)
  line L245 (-38.5, 44) -> (-41.5, 44)
  line L246 (-41.5, 44) -> (-41.5, -35.5244)
  line L247 (-35.5, 44) -> (-35.5, -38.6413)
  line L248 (27.5, 44) -> (27.5, -38.6413)
  line L249 (33.5, 44) -> (33.5, -35.5244)
  line L250 (-63, -2.4999) -> (-63, 44)
  line L251 (-63, 20.7501) -> (-63, 23.7501)
  line L252 (-63, 20.7501) -> (-63, 17.7501)
  line L253 (-63, 23.7501) -> (55, 23.7501)
  line L254 (-63, 17.7501) -> (55, 17.7501)
  line L255 (-41.5, -2.4999) -> (-35.5, -2.4999)
  line L256 (-28.25, -22.7914) -> (-63, -22.7914)
  line L257 (-28.25, -16.7914) -> (-63, -16.7914)
  line L258 (-28.25, -22.7914) -> (55, -22.7914)
  line L259 (-28.25, -16.7914) -> (55, -16.7914)
  line L260 (-14, -2.4999) -> (-24, -2.4999)
  line L261 (-24, -2.4999) -> (-24, -7.4999)
  line L262 (-24, -7.4999) -> (-14, -7.4999)
  line L263 (-14, -7.4999) -> (-14, -2.4999)
  line L264 (-14, -2.4999) -> (-24, -2.4999)
  line L265 (-24, -2.4999) -> (-24, 2.5001)
  line L266 (-24, 2.5001) -> (-14, 2.5001)
  line L267 (-14, 2.5001) -> (-14, -2.4999)
  line L268 (-24, -7.4999) -> (-14, -16.7914)
  line L269 (-24, 2.5001) -> (-14, 17.7501)
  line L270 (6, -2.4999) -> (16, -2.4999)
  line L271 (16, -2.4999) -> (16, -7.4999)
  line L272 (16, -7.4999) -> (6, -7.4999)
  line L273 (6, -7.4999) -> (6, -2.4999)
  line L274 (6, -2.4999) -> (16, -2.4999)
  line L275 (16, -2.4999) -> (16, 2.5001)
  line L276 (16, 2.5001) -> (6, 2.5001)
  line L277 (6, 2.5001) -> (6, -2.4999)
  line L278 (6, -16.7914) -> (16, -7.4999)
  line L279 (6, 17.7501) -> (16, 2.5001)
  circle A16 centre (-19, -2.4999) radius 1.65
  circle A17 centre (11, -2.4999) radius 1.65
  line L280 (31, 110) -> (37, 110)
  line L281 (37, 110) -> (37, 134)
  line L282 (37, 134) -> (31, 134)
  line L283 (31, 134) -> (31, 110)
  line L284 (-39, 110) -> (-45, 110)
  line L285 (-45, 110) -> (-45, 134)
  line L286 (-45, 134) -> (-39, 134)
  line L287 (-39, 134) -> (-39, 110)
  line L288 (-45, 134) -> (37, 134)
  line L289 (37, 134) -> (37, 128)
  line L290 (37, 128) -> (-45, 128)
  line L291 (-45, 128) -> (-45, 134)
  line L292 (-14, 50) -> (6, 50)
  line L293 (6, 50) -> (6, 134)
  line L294 (6, 134) -> (-14, 134)
  line L295 (-14, 134) -> (-14, 50)
  line L296 (-32, 110) -> (24, 110)
  line L297 (24, 110) -> (24, 104)
  line L298 (24, 104) -> (-32, 104)
  line L299 (-32, 104) -> (-32, 110)
  line L300 (-32, 50) -> (-32, 104)
  line L301 (-23, 77) -> (24, 77)
  line L302 (-23, 83) -> (24, 83)
  line L303 (-23, 77) -> (-32, 77)
  line L304 (-23, 83) -> (-32, 83)
  line L305 (15.25, 87.9939) -> (-45, 88)
  line L306 (15.25, 87.9939) -> (37, 88)
  line L307 (27, 55) -> (22, 55)
  line L308 (-35, 55) -> (-30, 55)
  line L309 (22, 55) -> (22, 50)
  line L310 (-30, 55) -> (-30, 50)
  line L311 (22, 55) -> (22, 104)
  line L312 (-30, 55) -> (-30, 104)
  line L313 (15.1097, -130.0661) -> (-8.0853, -133.5454)
  line L314 (15.1097, -130.0661) -> (31.1911, -127.6539)
  line L315 (-21.6529, -130.2847) -> (0.0848, -133.5454)
  line L316 (-32.9976, -128.0417) -> (-26.7328, -124)
  line L317 (24.997, -128.0416) -> (18.7323, -124)
  line L318 (24.997, -128.0416) -> (27.739, -129.8107)
  line L319 (-21.6529, -130.2847) -> (-37.3372, -127.9321)
  line L320 (-32.9976, -128.0417) -> (-37.6808, -131.063)
  line L321 (-1.0003, -135.9997) -> (-1.0003, -124)
  line L322 (-7.0003, -135.9997) -> (-7.0003, -124)
  dimension "d198" = 0
  dimension "d199" = -50
  dimension "d202" = 0
  dimension "d203" = -50
  dimension "d208" = 82
  dimension "d209" = 84
  dimension "d210" = 78
  dimension "d211" = 130
  dimension "d212" = 17
  dimension "d213" = 113
  dimension "d214" = 8
  dimension "d217" = 80
  dimension "d218" = 5
  dimension "d234" = 6
  dimension "d254" = 3.3
  dimension "d255" = 3.3
  dimension "d256" = 3.3
  dimension "d257" = 53
  dimension "d265" = 52
  dimension "d266" = 52
  dimension "d267" = 2.2
  dimension "d268" = 2.2
  dimension "d269" = 13
  dimension "d270" = 60
  dimension "d271" = 13
  dimension "d272" = 60
  dimension "d273" = 60
  dimension "d274" = 6
  dimension "d275" = 60
  dimension "d276" = 3
  dimension "d277" = 5
  dimension "d278" = 3.2
  dimension "d279" = 3
  dimension "d280" = 5
  dimension "d281" = 3.2
  dimension "d300" = 8
  dimension "d301" = 8
  dimension "d303" = 6
  dimension "d304" = 6
  dimension "d305" = 6
  dimension "d306" = 6
  dimension "d307" = 6
  dimension "d308" = 6
  dimension "d310" = 6
  dimension "d311" = 6
  dimension "d312" = 6
  dimension "d313" = 6
  dimension "d314" = 6
  dimension "d315" = 10
  dimension "d316" = 10
  dimension "d319" = 3
  dimension "d320" = 3
  dimension "d325" = 3
  dimension "d326" = 3
  dimension "d327" = 3
  dimension "d328" = 3
  dimension "d329" = 6
  dimension "d334" = 6
  dimension "d335" = 6
  dimension "d336" = 6
  dimension "d338" = 6
  dimension "d339" = 6
  dimension "d342" = 3
  dimension "d343" = 3
  dimension "d344" = 3
  dimension "d345" = 3
  dimension "d346" = 10
  dimension "d347" = 3
  dimension "d348" = 3
  dimension "d349" = 3
  dimension "d350" = 3
  dimension "d354" = 3
  dimension "d356" = 3
  dimension "d357" = 3
  dimension "d358" = 3
  dimension "d371" = 9
  dimension "d372" = 9
  dimension "d375" = 6
  dimension "d376" = 6
  dimension "d377" = 6
  dimension "d378" = 6
  dimension "d379" = 6
  dimension "d380" = 6
  dimension "d381" = 10
  dimension "d382" = 10
  dimension "d383" = 3
  dimension "d384" = 3
  dimension "d385" = 3
  dimension "d386" = 3
  dimension "d387" = 3
  dimension "d388" = 3
  dimension "d391" = 10
  dimension "d392" = 5
  dimension "d393" = 5
  dimension "d396" = 10
  dimension "d397" = 5
  dimension "d398" = 10
  dimension "d399" = 5
  dimension "d400" = 3.3
  dimension "d401" = 3.3
  dimension "d404" = 6
  dimension "d405" = 6
  dimension "d411" = 5
  dimension "d412" = 5
  constraint horizontal L9
  constraint vertical L29
  constraint horizontal L26
  constraint vertical L13
  constraint horizontal L14
  constraint vertical L2
  constraint vertical L1
  constraint horizontal L0
  constraint vertical L6
  constraint horizontal L5
  constraint vertical L4
  constraint horizontal L23
  constraint vertical L25
  constraint horizontal L22
  constraint vertical L51
  constraint vertical L8
  constraint vertical L54
  constraint vertical L34
  constraint horizontal L41
  constraint midpoint L16.start L5
  constraint perpendicular L15 L30
  constraint perpendicular L10 L30
  constraint coincident L10.end A3.centre
  constraint coincident A1.centre L15.end
  constraint horizontal L47
  constraint vertical L18
  constraint horizontal L36
  constraint vertical L17
  constraint horizontal L44
  constraint vertical L24
  constraint horizontal L33
  constraint vertical L11
  constraint horizontal L49
  constraint vertical L20
  constraint horizontal L37
  constraint vertical L27
  constraint horizontal L46
  constraint vertical L28
  constraint horizontal L19
  constraint vertical L32
  constraint horizontal L45
  constraint vertical L38
  constraint horizontal L43
  constraint vertical L50
  constraint coincident L38.end L43.start
  constraint horizontal L48
  constraint vertical L35
  constraint horizontal L39
  constraint vertical L42
  constraint coincident L35.end L39.start
  constraint horizontal L55
  constraint vertical L56
  constraint horizontal L57
  constraint vertical L58
  constraint horizontal L63
  constraint vertical L64
  constraint horizontal L65
  constraint vertical L66
  constraint horizontal L67
  constraint vertical L68
  constraint horizontal L69
  constraint vertical L70
  constraint coincident L62 L71.start
  constraint perpendicular L62 L71
  constraint midpoint L62 L72.start
  constraint perpendicular L62 L72
  constraint horizontal L73
  constraint vertical L74
  constraint horizontal L75
  constraint vertical L76
  constraint horizontal L77
  constraint vertical L78
  constraint horizontal L79
  constraint vertical L80
  constraint coincident L68 L81.end
  constraint perpendicular L72 L81
  constraint horizontal L82
  constraint vertical L83
  constraint horizontal L84
  constraint vertical L85
  constraint coincident L61 L86.start
  constraint perpendicular L61 L86
  constraint coincident L64 L87.end
  constraint perpendicular L86 L87
  constraint coincident L84 L88.end
  constraint perpendicular L71 L88
  constraint horizontal L89
  constraint vertical L90
  constraint horizontal L91
  constraint vertical L92
  constraint coincident L21 L93.start
  constraint perpendicular L21 L93
  constraint coincident L31 L94.start
  constraint perpendicular L31 L94
  constraint coincident L21 L95.start
  constraint perpendicular L21 L95
  constraint coincident L31 L96.start
  constraint perpendicular L31 L96
  constraint coincident L91 L99.end
  constraint perpendicular L94 L99
  constraint coincident L64 L100.end
  constraint perpendicular L93 L100
  constraint coincident L91 L101.end
  constraint perpendicular L95 L101
  constraint coincident L68 L102.end
  constraint perpendicular L96 L102
  constraint concentric A2 A13
  constraint concentric A12 A14
  constraint horizontal L103
  constraint vertical L104
  constraint horizontal L105
  constraint vertical L106
  constraint coincident A14 L108.start
  constraint coincident L107 L108.start
  constraint coincident L102 L108.end
  constraint tangent A14 L108
  constraint perpendicular L107 L108
  constraint coincident L107 L109.start
  constraint coincident A14 L109.start
  constraint coincident L98 L109.end
  constraint tangent A14 L109
  constraint midpoint L103 L110.start
  constraint parallel L103 L110
  constraint parallel L110 L111
  constraint perpendicular L103 L112
  constraint coincident L81 L113.end
  constraint perpendicular L103 L113
  constraint horizontal L114
  constraint vertical L115
  constraint horizontal L116
  constraint vertical L117
  constraint coincident A13 L119.start
  constraint coincident L118 L119.start
  constraint coincident L100 L119.end
  constraint tangent A13 L119
  constraint perpendicular L118 L119
  constraint coincident A13 L120.start
  constraint coincident L118 L120.start
  constraint coincident L101 L120.end
  constraint tangent A13 L120
  constraint midpoint L114 L121.start
  constraint parallel L114 L121
  constraint parallel L114 L122
  constraint perpendicular L122 L123
  constraint perpendicular L121 L124
  constraint horizontal L125
  constraint vertical L126
  constraint horizontal L127
  constraint vertical L128
  constraint midpoint L55 L125.start
  constraint horizontal L129
  constraint vertical L130
  constraint horizontal L131
  constraint vertical L132
  constraint horizontal L133
  constraint vertical L134
  constraint horizontal L135
  constraint vertical L136
  constraint horizontal L137
  constraint vertical L138
  constraint horizontal L139
  constraint vertical L140
  constraint horizontal L141
  constraint vertical L142
  constraint horizontal L143
  constraint vertical L144
  constraint horizontal L145
  constraint vertical L146
  constraint horizontal L147
  constraint vertical L148
  constraint midpoint L0 L149.start
  constraint coincident L151 L152.start
  constraint perpendicular L151 L152
  constraint perpendicular L151 L153
  constraint coincident L5 L154.end
  constraint perpendicular L152 L154
  constraint coincident L142 L155.end
  constraint perpendicular L153 L155
  constraint coincident L0 L156.end
  constraint perpendicular L153 L156
  constraint perpendicular L152 L157
  constraint coincident L158 L159.start
  constraint perpendicular L158 L159
  constraint perpendicular L158 L160
  constraint coincident L5 L161.end
  constraint perpendicular L160 L161
  constraint coincident L146 L162.end
  constraint perpendicular L159 L162
  constraint coincident L0 L163.end
  constraint perpendicular L159 L163
  constraint perpendicular L160 L164
  constraint concentric A0 A15
  constraint midpoint L84 L165.start
  constraint coincident L165 L167.start
  constraint perpendicular L165 L167
  constraint coincident L165 L168.start
  constraint perpendicular L165 L168
  constraint coincident L84 L169.end
  constraint perpendicular L168 L169
  constraint perpendicular L167 L170
  constraint coincident L91 L171.end
  constraint perpendicular L167 L171
  constraint coincident L101 L172.end
  constraint perpendicular L168 L172
  constraint coincident L166 L173.start
  constraint perpendicular L166 L173
  constraint coincident L166 L174.start
  constraint perpendicular L166 L174
  constraint coincident L91 L176.end
  constraint perpendicular L174 L176
  constraint coincident L84 L177.end
  constraint perpendicular L173 L177
  constraint coincident L99 L178.end
  constraint perpendicular L173 L178
  constraint perpendicular L72 L180
  constraint midpoint L179 L181.start
  constraint coincident L178 L181.end
  constraint perpendicular L178 L181
  constraint coincident L181 L182.start
  constraint perpendicular L181 L182
  constraint coincident L179 L183.end
  constraint perpendicular L182 L183
  constraint coincident L178 L184.end
  constraint perpendicular L178 L184
  constraint perpendicular L86 L185
  constraint coincident L84 L186.end
  constraint parallel L185 L186
  constraint midpoint L186 L187.start
  constraint coincident L169 L187.end
  constraint perpendicular L169 L187
  constraint coincident L187 L188.start
  constraint perpendicular L187 L188
  constraint perpendicular L187 L189
  constraint coincident L186 L190.end
  constraint perpendicular L189 L190
  constraint coincident L186 L191.end
  constraint perpendicular L188 L191
  constraint coincident L169 L192.end
  constraint perpendicular L169 L192
  constraint coincident L169 L193.end
  constraint perpendicular L169 L193
  constraint coincident L181 L194.start
  constraint perpendicular L181 L194
  constraint perpendicular L194 L195
  constraint coincident L177 L196.end
  constraint perpendicular L177 L196
  constraint coincident A13 L197.end
  constraint perpendicular L10 L197
  constraint coincident A13 L198.end
  constraint perpendicular L114 L198
  constraint coincident A14 L199.end
  constraint perpendicular L103 L199
  constraint coincident A14 L200.end
  constraint perpendicular L103 L200
  constraint coincident L175 L202.end
  constraint coincident L22 L202.end
  constraint coincident L22 L203.end
  constraint coincident L166 L203.end
  constraint horizontal L205
  constraint vertical L206
  constraint horizontal L207
  constraint vertical L208
  constraint horizontal L209
  constraint vertical L210
  constraint horizontal L211
  constraint vertical L212
  constraint horizontal L213
  constraint vertical L214
  constraint horizontal L215
  constraint vertical L216
  constraint horizontal L217
  constraint vertical L218
  constraint horizontal L219
  constraint vertical L220
  constraint coincident L7 L221.start
  constraint perpendicular L7 L221
  constraint coincident L7 L222.start
  constraint perpendicular L7 L222
  constraint coincident L139 L224.end
  constraint perpendicular L222 L224
  constraint coincident L214 L225.end
  constraint perpendicular L221 L225
  constraint coincident L3 L226.start
  constraint perpendicular L3 L226
  constraint coincident L218 L227.end
  constraint perpendicular L226 L227
  constraint coincident L139 L228.end
  constraint perpendicular L226 L228
  constraint horizontal L229
  constraint vertical L230
  constraint horizontal L231
  constraint vertical L232
  constraint horizontal L233
  constraint vertical L234
  constraint horizontal L235
  constraint midpoint L139 L233.start
  constraint horizontal L236
  constraint vertical L237
  constraint horizontal L238
  constraint coincident L1 L239.start
  constraint coincident L220 L239.end
  constraint perpendicular L220 L239
  constraint coincident L214 L240.end
  constraint coincident L231 L240.end
  constraint perpendicular L214 L240
  constraint coincident L218 L241.end
  constraint coincident L231 L241.end
  constraint perpendicular L218 L241
  constraint midpoint L240 L244.start
  constraint midpoint L241 L242.start
  constraint coincident L224 L246.end
  constraint perpendicular L231 L246
  constraint coincident L224 L247.end
  constraint perpendicular L240 L247
  constraint coincident L228 L248.end
  constraint perpendicular L231 L248
  constraint coincident L228 L249.end
  constraint perpendicular L231 L249
  constraint coincident L214 L250.start
  constraint coincident L239 L250.start
  constraint midpoint L250 L251.start
  constraint coincident L218 L253.end
  constraint perpendicular L218 L253
  constraint coincident L218 L254.end
  constraint perpendicular L218 L254
  constraint coincident L246 L255.start
  constraint coincident L239 L255.start
  constraint coincident L239 L255.end
  constraint coincident L247 L255.end
  constraint coincident L214 L256.end
  constraint perpendicular L214 L256
  constraint coincident L214 L257.end
  constraint perpendicular L214 L257
  constraint coincident L218 L258.end
  constraint perpendicular L218 L258
  constraint coincident L218 L259.end
  constraint perpendicular L218 L259
  constraint horizontal L260
  constraint vertical L261
  constraint horizontal L262
  constraint vertical L263
  constraint coincident L239 L260.start
  constraint coincident L234 L260.start
  constraint horizontal L264
  constraint vertical L265
  constraint horizontal L266
  constraint vertical L267
  constraint coincident L234 L268.end
  constraint coincident L234 L269.end
  constraint coincident L254 L269.end
  constraint horizontal L270
  constraint vertical L271
  constraint horizontal L272
  constraint vertical L273
  constraint coincident L237 L270.start
  constraint coincident L239 L270.start
  constraint horizontal L274
  constraint vertical L275
  constraint horizontal L276
  constraint vertical L277
  constraint coincident L259 L278.start
  constraint coincident L237 L278.start
  constraint coincident L237 L279.start
  constraint coincident L254 L279.start
  constraint midpoint L264 A16.centre
  constraint midpoint L270 A17.centre
  constraint horizontal L280
  constraint vertical L281
  constraint horizontal L282
  constraint vertical L283
  constraint horizontal L284
  constraint vertical L285
  constraint horizontal L286
  constraint vertical L287
  constraint horizontal L288
  constraint vertical L289
  constraint horizontal L290
  constraint vertical L291
  constraint horizontal L292
  constraint vertical L293
  constraint horizontal L294
  constraint coincident L26 L293.end
  constraint coincident L9 L292.start
  constraint horizontal L296
  constraint vertical L297
  constraint horizontal L298
  constraint vertical L299
  constraint coincident L18 L301.end
  constraint perpendicular L18 L301
  constraint coincident L18 L302.end
  constraint perpendicular L18 L302
  constraint midpoint L300 L303.end
  constraint coincident L300 L304.end
  constraint coincident L11 L305.end
  constraint coincident L17 L306.end
  constraint coincident A8.centre L307.start
  constraint horizontal L307
  constraint coincident A4.centre L308.start
  constraint horizontal L308
  constraint coincident L229 L309.end
  constraint perpendicular L229 L309
  constraint coincident L9 L310.end
  constraint coincident L14 L310.end
  constraint coincident L298 L311.end
  constraint perpendicular L298 L311
  constraint coincident L298 L312.end
  constraint perpendicular L298 L312